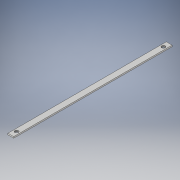
# Autodesk Inventor part: Pedal Bar
Saved by Autodesk Inventor 2019 (Build 230136000, 136)
## iProperties
Created: 2020-06-01
Part Number: Pedal Bar
Material: Generic
Document SubType Name: Modeling
Designer: 18186
Density: 1 g/cm^3
Appearance: Default
Author: 18186
Autodesk Inventor part; units mm, degrees
ref_plane "YZ Plane" through (0, 0, 0) normal (1, 0, 0) x (0, 1, 0)
ref_plane "XZ Plane" through (0, 0, 0) normal (0, 1, 0) x (-1, 0, 0)
ref_plane "XY Plane" through (0, 0, 0) normal (0, 0, 1) x (1, 0, 0)
sketch "Sketch1" plane through (0, 0, 0) normal (0, 0, 1) x (1, 0, 0)
  line L0 (2.54, -0.635) -> (-2.54, -0.635)
  line L1 (-2.54, -0.635) -> (-2.54, 0.635)
  line L2 (-2.54, 0.635) -> (2.54, 0.635)
  line L3 (2.54, 0.635) -> (2.54, -0.635)
  line L4 (2.54, -0.635) -> (-2.54, 0.635) construction
  line L5 (-2.54, -0.635) -> (2.54, 0.635) construction
  point P0 (0, 0)
  dimension "d0" = 5.08
  dimension "d1" = 1.27
  constraints: 12 end point, 2 midpoint, 2 parallel, 1 horizontal, 1 perpendicular
  measures "d0" distance of L1.end L2.end
  measures "d1" distance of L0.end L1.end
extrude "Extrusion1" add sketch "Sketch1" along normal blind 119.38
ref_plane "Work Plane1" through (0, 0, 59.69) normal (0, 0, 1) x (1, 0, 0)
sketch "Sketch2" plane through (0, 0, 119.38) normal (0, 0, 1) x (1, 0, 0)
  line L0 (2.54, 0.635) -> (-2.54, 0.635) projected
  line L1 (-2.54, 0.635) -> (-2.54, -0.635) projected
  line L2 (-2.54, -0.635) -> (2.54, -0.635) projected
  line L3 (2.54, -0.635) -> (2.54, 0.635) projected
  point P0 (0, 0)
extrude "Extrusion2" add sketch "Sketch2" along normal blind 10.16
sketch "Sketch3" plane through (-2.54, 0.635, 0) normal (0, 1, 0) x (1, 0, 0)
  line L0 (5.08, -119.38) -> (0, -119.38) construction
  line L1 (2.54, -119.38) -> (2.54, -129.54) construction
  line L2 (0, -129.54) -> (5.08, -129.54) construction
  circle A0 centre (2.54, -124.46) radius 1.5875
  point P0 (2.54, 0)
  dimension "d6" = 3.175
  constraints: 3 midpoint, 2 end point, 1 centre point
  measures "d6" diameter of A0
extrude "Extrusion3" cut sketch "Sketch3" against normal blind 6.35
mirror "Mirror1" about plane through (0, 0, 59.69) normal (0, 0, 1) of "Extrusion2"
mirror "Mirror2" about plane through (0, 0, 59.69) normal (0, 0, 1) of "Extrusion3"
thread "Thread1" size "5-40 UNC" class "2B" standard "ANSI Unified Screw Threads" full length
thread "Thread2" size "5-40 UNC" class "2B" standard "ANSI Unified Screw Threads" full length
body "Solid1"
